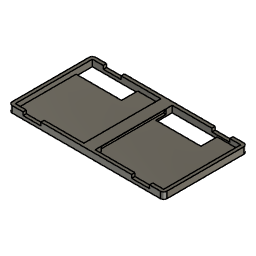
Top Center Cover 2x1 v7 (Autodesk Fusion 360 design; units mm, degrees)
Autodesk Fusion 360 part; units mm, degrees
note: some values were not read from the file. Set by a fixed rule: which sketch regions a step uses.
sketch "Schizzo1" plane through (0, 0, 0) normal (0, 0, 1) x (1, 0, 0)
  line L0 (64.6508, 75.5456) -> (160.3508, 75.5456) construction
  line L1 (160.3508, 75.5456) -> (160.3508, 23.8456) construction
  line L2 (160.3508, 23.8456) -> (64.6508, 23.8456) construction
  line L3 (64.6508, 23.8456) -> (64.6508, 75.5456) construction
  line L4 (64.6508, 49.6956) -> (160.3508, 49.6956) construction
  line L5 (112.5008, 75.5456) -> (112.5008, 23.8456) construction
  line L6 (160.2508, 23.9456) -> (64.7508, 23.9456)
  line L7 (64.7508, 23.9456) -> (64.7508, 75.4456)
  line L8 (64.7508, 75.4456) -> (160.2508, 75.4456)
  line L9 (160.2508, 75.4456) -> (160.2508, 23.9456)
  line L10 (160.2508, 23.9456) -> (64.7508, 75.4456) construction
  line L11 (64.7508, 23.9456) -> (160.2508, 75.4456) construction
  line L12 (146.3653, 67.9576) -> (78.6363, 31.4336) construction
  line L13 (78.6363, 67.9576) -> (146.3653, 31.4336) construction
  point P0 (112.5008, 49.6956)
  point P1 (112.5008, 49.6956)
  dimension "d1" = 95.7
  dimension "d2" = 51.7
  dimension "d3" = 0.1
  dimension "d4" = 0.1
  constraint horizontal L0
  constraint vertical L1
  constraint horizontal L2
  constraint vertical L3
  constraint midpoint L3 L4.start
  constraint midpoint L1 L4.end
  constraint midpoint L0 L5.start
  constraint midpoint L2 L5.end
  constraint horizontal L6
  constraint perpendicular L6 L7
  constraint parallel L6 L8
  constraint parallel L7 L9
  constraint coincident L10 P1
  constraint coincident L11 P1
  constraint midpoint L4 P1
  constraint coincident L12 P1
  constraint coincident L13 P1
  constraint coincident L11 L12.start
  constraint coincident P1 P0
  measures "d1" distance of L0.start L0.end
  measures "d2" distance of L0.start L2.end
  measures "d3" distance of L3 L7
  measures "d4" distance of L0 L8
extrude "Estrusione1" add sketch "Schizzo1" along normal blind 4
fillet "Raccordo1" radius 2 4 edges at (64.7508, 23.9456, 2) (64.7508, 75.4456, 2) (160.2508, 23.9456, 2) (160.2508, 75.4456, 2)
sketch "Schizzo2" plane through (0, 0, 4) normal (0, 0, 1) x (-1, 0, 0)
  arc A0 (-160.2508, -73.4456) -> (-158.2508, -75.4456) centre (-158.2508, -73.4456) ccw
  line L0 (-158.2508, -75.4456) -> (-66.7508, -75.4456)
  arc A1 (-66.7508, -75.4456) -> (-64.7508, -73.4456) centre (-66.7508, -73.4456) ccw
  line L1 (-64.7508, -73.4456) -> (-64.7508, -25.9456)
  arc A2 (-64.7508, -25.9456) -> (-66.7508, -23.9456) centre (-66.7508, -25.9456) ccw
  line L2 (-66.7508, -23.9456) -> (-158.2508, -23.9456)
  arc A3 (-158.2508, -23.9456) -> (-160.2508, -25.9456) centre (-158.2508, -25.9456) ccw
  line L3 (-160.2508, -25.9456) -> (-160.2508, -73.4456)
  line L4 (-64.7508, -75.4456) -> (-160.2508, -75.4456) construction
  line L5 (-160.2508, -75.4456) -> (-160.2508, -23.9456) construction
  line L6 (-160.2508, -23.9456) -> (-64.7508, -23.9456) construction
  line L7 (-64.7508, -23.9456) -> (-64.7508, -75.4456) construction
  line L8 (-64.7508, -49.6956) -> (-160.2508, -49.6956) construction
  line L9 (-112.5008, -75.4456) -> (-112.5008, -23.9456) construction
  line L10 (-158.2508, -73.4456) -> (-66.7508, -73.4456)
  line L11 (-66.7508, -73.4456) -> (-66.7508, -25.9456)
  line L12 (-66.7508, -25.9456) -> (-158.2508, -25.9456)
  line L13 (-158.2508, -25.9456) -> (-158.2508, -73.4456)
  line L14 (-158.2508, -73.4456) -> (-66.7508, -25.9456) construction
  line L15 (-66.7508, -73.4456) -> (-158.2508, -25.9456) construction
  line L16 (-116.0008, -25.9456) -> (-109.0008, -25.9456)
  line L17 (-109.0008, -25.9456) -> (-109.0008, -73.4456)
  line L18 (-109.0008, -73.4456) -> (-116.0008, -73.4456)
  line L19 (-116.0008, -73.4456) -> (-116.0008, -25.9456)
  line L20 (-116.0008, -25.9456) -> (-109.0008, -73.4456) construction
  line L21 (-109.0008, -25.9456) -> (-116.0008, -73.4456) construction
  line L22 (-84.5008, -72.4456) -> (-73.5008, -72.4456)
  line L23 (-73.5008, -72.4456) -> (-73.5008, -75.4456)
  line L24 (-73.5008, -75.4456) -> (-84.5008, -75.4456)
  line L25 (-84.5008, -75.4456) -> (-84.5008, -72.4456)
  line L26 (-84.5008, -72.4456) -> (-73.5008, -75.4456) construction
  line L27 (-73.5008, -72.4456) -> (-84.5008, -75.4456) construction
  line L28 (-151.5008, -72.4456) -> (-151.5008, -75.4456)
  line L29 (-151.5008, -75.4456) -> (-140.5008, -75.4456)
  line L30 (-140.5008, -72.4456) -> (-151.5008, -72.4456)
  line L31 (-140.5008, -75.4456) -> (-140.5008, -72.4456)
  line L32 (-151.5008, -72.4456) -> (-140.5008, -75.4456) construction
  line L33 (-140.5008, -72.4456) -> (-151.5008, -75.4456) construction
  line L34 (-66.7508, -73.4456) -> (-94.7508, -73.4456)
  line L35 (-94.7508, -73.4456) -> (-94.7508, -63.4456)
  line L36 (-94.7508, -63.4456) -> (-66.7508, -63.4456)
  line L37 (-66.7508, -63.4456) -> (-66.7508, -73.4456)
  line L38 (-115.7508, -73.4456) -> (-143.7508, -73.4456)
  line L39 (-143.7508, -73.4456) -> (-143.7508, -63.4456)
  line L40 (-143.7508, -63.4456) -> (-115.7508, -63.4456)
  line L41 (-115.7508, -63.4456) -> (-115.7508, -73.4456)
  line L42 (-84.5008, -26.9456) -> (-73.5008, -26.9456)
  line L43 (-73.5008, -26.9456) -> (-73.5008, -23.9456)
  line L44 (-73.5008, -23.9456) -> (-84.5008, -23.9456)
  line L45 (-84.5008, -23.9456) -> (-84.5008, -26.9456)
  line L46 (-140.5008, -26.9456) -> (-151.5008, -26.9456)
  line L47 (-140.5008, -23.9456) -> (-140.5008, -26.9456)
  line L48 (-151.5008, -26.9456) -> (-151.5008, -23.9456)
  line L49 (-151.5008, -23.9456) -> (-140.5008, -23.9456)
  point P0 (-112.5008, -49.6956)
  point P1 (-112.5008, -49.6956)
  point P2 (-79.0008, -73.9456)
  point P3 (-146.0008, -73.9456)
  dimension "d9" = 2
  dimension "d10" = 2
  dimension "d11" = 7
  dimension "d14" = 11
  dimension "d15" = 3
  dimension "d16" = 67
  dimension "d19" = 28
  dimension "d20" = 10
  dimension "d21" = 28
  dimension "d22" = 10
  dimension "d23" = 49
  constraint horizontal L4
  constraint vertical L5
  constraint horizontal L6
  constraint vertical L7
  constraint collinear L1 L7
  constraint collinear L0 L4
  constraint collinear L3 L5
  constraint collinear L2 L6
  constraint midpoint L7 L8.start
  constraint midpoint L5 L8.end
  constraint midpoint L0 L9.start
  constraint midpoint L6 L9.end
  constraint horizontal L10
  constraint perpendicular L10 L11
  constraint parallel L10 L12
  constraint parallel L11 L13
  constraint coincident L14 P1
  constraint coincident L15 P1
  constraint midpoint L9 P1
  constraint horizontal L16
  constraint perpendicular L16 L17
  constraint parallel L16 L18
  constraint parallel L17 L19
  constraint coincident L20 P1
  constraint coincident L21 P1
  constraint coincident P1 P0
  constraint collinear L10 L18
  constraint horizontal L22
  constraint perpendicular L22 L23
  constraint parallel L22 L24
  constraint parallel L23 L25
  constraint coincident L26 P2
  constraint coincident L27 P2
  constraint symmetric L9 L22.start L30.start
  constraint symmetric L9 L22.end L28.start
  constraint symmetric L9 L23.end L28.end
  constraint symmetric L9 L24.end L29.end
  constraint symmetric L9 P2 P3
  constraint collinear L4 L24
  constraint horizontal L34
  constraint vertical L35
  constraint horizontal L36
  constraint vertical L37
  constraint coincident A1.centre L10.end
  constraint horizontal L38
  constraint vertical L39
  constraint horizontal L40
  constraint vertical L41
  constraint collinear L10 L38
  constraint symmetric L8 L22.start L42.start
  constraint symmetric L8 L22.end L42.end
  constraint symmetric L8 L23.end L43.end
  constraint symmetric L8 L24.end L44.end
  constraint symmetric L8 L28.start L46.end
  constraint symmetric L8 L28.end L48.end
  constraint symmetric L8 L29.end L47.start
  constraint symmetric L8 L30.start L46.start
  measures "d9" distance of L7 L11
  measures "d10" distance of L4 L10
  measures "d11" distance of L17.end L18.end
  measures "d14" distance of L23.end L24.end
  measures "d15" distance of L22.end L23.end
  measures "d16" distance of P2 P3
  measures "d19" distance of A1.centre L34.end
  measures "d20" distance of A1.centre L36.end
  measures "d21" distance of L39 L41
  measures "d22" distance of L38 L40
  measures "d23" distance of L35 L39
extrude "Estrusione2" cut sketch "Schizzo2" against normal blind 3 contours L10 L28 L30 L39 | L10 L12 L13 L19 L28 L30 L39 L40 L46 L47 L48 | L10 L19 L30 L31 L38 L39 L40 | L10 L30 L31 L38 L39 | L12 L46 L47 L48 | L10 L22 L23 L25 L34 | L10 L11 L22 L23 L25 L34 L35 L36 L37 | L10 L11 L12 L17 L35 L36 L42 L43 L45 | L12 L42 L43 L45
extrude "Estrusione4" cut sketch "Schizzo2" against normal blind 4 contours L10 L19 L30 L31 L38 L39 L40 | L10 L30 L31 L38 L39 | L10 L22 L23 L25 L34 | L10 L11 L22 L23 L25 L34 L35 L36 L37
extrude "Estrusione5" cut sketch "Schizzo2" against normal blind 2 contours L0 L10 L28 L29 L31 L38 | L2 L12 L47 L48 L49 | L0 L10 L23 L24 L25 L34 | L2 L12 L43 L44 L45
ref_plane "Piano di lavoro1" through (112.5008, 49.6956, 4) normal (0, -1, 0) x (1, 0, 0)
sketch "Schizzo3" plane through (0, 49.6956, 0) normal (0, -1, 0) x (-1, 0, 0)
  line L0 (-64.7508, -4) -> (-160.3508, -4) construction
  line L1 (-160.3508, -4) -> (-160.3508, 0) construction
  line L2 (-160.3508, 0) -> (-64.7508, 0) construction
  line L3 (-64.7508, 0) -> (-64.7508, -4) construction
  line L4 (-109.0008, -1) -> (-109.0008, -4) construction
  line L5 (-64.7508, -1) -> (-160.3508, -1) construction
  line L6 (-94.7508, -1) -> (-109.0008, -1) construction
  line L7 (-109.0008, -4) -> (-109.0008, 0) construction
  line L8 (-116, -4) -> (-116, 0) construction
  line L9 (-109.0008, -1) -> (-109.0008, -4)
  line L10 (-109.0008, -4) -> (-110.7329, -1)
  line L11 (-110.7329, -1) -> (-109.0008, -1)
  line L12 (-110.7329, -1) -> (-109.0008, -4)
  line L13 (-109.0008, -4) -> (-109.0008, -1)
  line L14 (-112.5508, -4) -> (-112.5508, 0) construction
  line L15 (-116.1008, -4) -> (-114.3688, -1)
  line L16 (-116.1008, -4) -> (-116.1008, 0) construction
  line L17 (-114.3688, -1) -> (-116.1008, -1)
  line L18 (-116.1008, -4) -> (-116.1008, -1)
  point P0 (-64.7508, -4)
  point P1 (-160.3508, 0)
  point P2 (-109.0008, -4)
  dimension "d29" = 30
  constraint horizontal L0
  constraint vertical L1
  constraint horizontal L2
  constraint vertical L3
  constraint coincident P0 L0.start
  constraint coincident P1 L1.end
  constraint coincident L0 P2
  constraint perpendicular L0 L4
  constraint coincident L3 L5.start
  constraint coincident L1 L5.end
  constraint perpendicular L1 L5
  constraint collinear L5 L6
  constraint coincident L2 L7.end
  constraint perpendicular L2 L7
  constraint coincident L0 L8.start
  constraint coincident L2 L8.end
  constraint perpendicular L2 L8
  constraint coincident L5 L10.end
  constraint coincident L4.start L6.end
  constraint midpoint L0 L14.start
  constraint midpoint L2 L14.end
  constraint symmetric P2 L14 L15.start
  constraint symmetric L7.end L14 L16.end
  constraint symmetric L10.end L14 L15.end
  constraint symmetric L4.start L14 L17.end
  constraint coincident P2 L4.end
  measures "d29" angle of L9 L10
extrude "Estrusione6" cut sketch "Schizzo3" along normal mid plane 40
equation "d21 = d19"
equation "d22 = d20"
